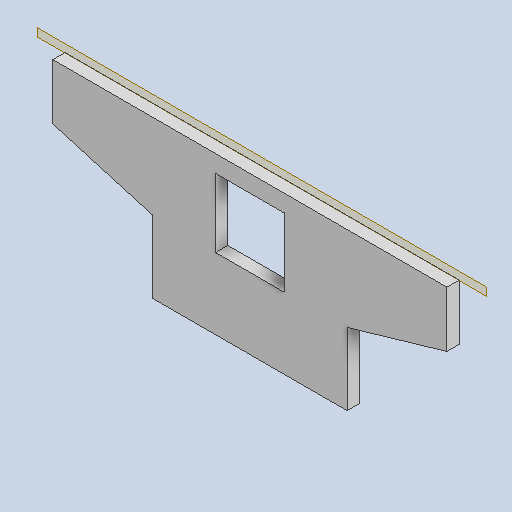
# Autodesk Inventor part: headstage_cap_top_closure
Saved by Autodesk Inventor 2023.4 (Build 274418000, 418)
## iProperties
Created: 2023-05-02
Part Number: headstage_cap_top_closure
Material: Generic
Document SubType Name: Modeling
Designer: mmelin
Density: 1 g/cm^3
Appearance: Default
Author: mmelin
Autodesk Inventor part; units mm, degrees
ref_plane "YZ Plane" through (0, 0, 0) normal (1, 0, 0) x (0, 1, 0)
ref_plane "XZ Plane" through (0, 0, 0) normal (0, 1, 0) x (-1, 0, 0)
ref_plane "XY Plane" through (0, 0, 0) normal (0, 0, 1) x (1, 0, 0)
ref_plane "Work Plane1" through (0, 0, 0) normal (0, 0, 1) x (1, 0, 0)
sketch "Sketch1" plane through (0, 0, 0) normal (0, 0, 1) x (1, 0, 0)
  line L0 (-16.7058, 0.002) -> (-16.7058, -2.798) projected
  line L1 (-12.6264, -3.9858) -> (-16.7058, -2.798) projected
  line L2 (-12.6264, -3.9858) -> (-12.6264, -7.006) projected
  line L3 (-4.0852, -7.006) -> (-4.0852, -3.9858) projected
  line L4 (-0.0058, -2.798) -> (-4.0852, -3.9858) projected
  line L5 (-0.0058, 0.002) -> (-0.0058, -2.798) projected
  line L6 (-16.7058, 0.002) -> (-0.0058, 0.002) projected
  line L7 (-4.0852, -7.006) -> (-12.6264, -7.006) projected
  line L8 (-16.4058, -0.298) -> (-0.3058, -0.298)
  line L9 (-0.3058, -0.298) -> (-0.3058, -2.5729)
  line L10 (-0.3058, -2.5729) -> (-4.3852, -3.7607)
  line L11 (-4.3852, -3.7607) -> (-4.3852, -6.706)
  line L12 (-4.3852, -6.706) -> (-12.3264, -6.706)
  line L13 (-12.3264, -6.706) -> (-12.3264, -3.7607)
  line L14 (-12.3264, -3.7607) -> (-16.4058, -2.5729)
  line L15 (-16.4058, -2.5729) -> (-16.4058, -0.298)
  line L16 (-2.523, -0.298) -> (-2.523, 0.002) construction
  line L17 (-16.4058, -0.4626) -> (-16.7058, -0.4626) construction
  line L18 (-6.5787, -6.706) -> (-6.5787, -7.006) construction
  line L19 (-0.3058, -0.7097) -> (-0.0058, -0.7097) construction
  line L20 (-2.0075, -3.0684) -> (-1.9236, -3.3564) construction
  line L21 (-13.1905, -3.5091) -> (-13.2743, -3.7971) construction
  line L22 (-12.3264, -6.0147) -> (-12.6264, -6.0147) construction
  line L23 (-4.3852, -6.1814) -> (-4.0852, -6.1814) construction
  line L24 (-9.7558, -0.998) -> (-6.9558, -0.998)
  line L25 (-6.9558, -0.998) -> (-6.9558, -3.798)
  line L26 (-6.9558, -3.798) -> (-9.7558, -3.798)
  line L27 (-9.7558, -3.798) -> (-9.7558, -0.998)
  line L28 (-9.7558, -1.5221) -> (-16.4058, -1.5221) construction
  line L29 (-0.3058, -1.3283) -> (-6.9558, -1.3283) construction
  point P0 (0, 0)
  dimension "d0" = 0.3
  dimension "d3" = 2.8
  dimension "d4" = 2.8
  dimension "d5" = 1
  constraints: 44 end point, 20 point on line, 13 perpendicular, 11 parallel, 8 equal length, 1 horizontal, 1 vertical
  measures "d0" distance of L16.start L16.end
  measures "d3" distance of L24.start L24.end
  measures "d4" distance of L26.end L24.start
  measures "d5" distance between parallel lines of L6 L24
extrude "Extrusion1" add sketch "Sketch1" along normal blind 0.5 contours L8 L9 L10 L11 L12 L13 L14 L15
body "Solid1"
